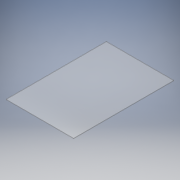
# Autodesk Inventor part: ElectricalBoard.ver1-1111-2019
Saved by Autodesk Inventor 2018 (Build 220112000, 112)
## iProperties
Created: 2019-11-12
Part Number: ElectricalBoard.ver1-1111-2019
Material: Polycarbonate, Clear
Document SubType Name: Modeling
Designer: JMHal
Density: 1.2 g/cm^3
Appearance: Polycarbonate - Clear
Author: JMHal
Autodesk Inventor part; units mm, degrees
ref_plane "YZ Plane" through (0, 0, 0) normal (1, 0, 0) x (0, 1, 0)
ref_plane "XZ Plane" through (0, 0, 0) normal (0, 1, 0) x (-1, 0, 0)
ref_plane "XY Plane" through (0, 0, 0) normal (0, 0, 1) x (1, 0, 0)
sketch "Sketch1" plane through (0, 0, 0) normal (0, 1, 0) x (-1, 0, 0)
  line L0 (0, 0) -> (393.7, 0)
  line L1 (393.7, 0) -> (393.7, -584.2)
  line L2 (393.7, -584.2) -> (0, -584.2)
  line L3 (0, -584.2) -> (0, 0)
  dimension "d0" = 393.7
  dimension "d1" = 584.2
  constraints: 8 end point, 2 parallel, 1 horizontal, 1 perpendicular
  measures "d0" distance of L1.end L2.end
  measures "d1" distance of L0.end L1.end
extrude "Extrusion1" add sketch "Sketch1" along normal blind 3.175
body "Solid1"
